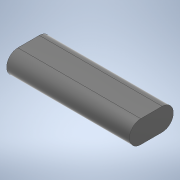
# Autodesk Inventor part: HX-2000MHT
Saved by Autodesk Inventor 2020 (Build 240168000, 168)
## iProperties
Created: 2019-11-07
Part Number: HX-2000MHT
Material: Generic
Document SubType Name: Modeling
Designer: maste
Density: 1 g/cm^3
Appearance: Smooth - Black
Author: maste
Autodesk Inventor part; units mm, degrees
ref_plane "YZ Plane" through (0, 0, 0) normal (1, 0, 0) x (0, 1, 0)
ref_plane "XZ Plane" through (0, 0, 0) normal (0, 1, 0) x (-1, 0, 0)
ref_plane "XY Plane" through (0, 0, 0) normal (0, 0, 1) x (1, 0, 0)
sketch "Sketch1" plane through (0, 0, 0) normal (1, 0, 0) x (0, 1, 0)
  line L0 (0, 0) -> (0, -46.5) construction
  line L1 (-11.9, -11.9) -> (-11.9, -34.6)
  line L2 (11.9, -34.6) -> (11.9, -11.9)
  arc A0 (11.9, -11.9) -> (-11.9, -11.9) centre (0, -11.9) ccw
  arc A1 (-11.9, -34.6) -> (11.9, -34.6) centre (0, -34.6) ccw
  point P0 (0, -23.25)
  dimension "d0" = 46.5
  dimension "d1" = 23.8
  constraints: 8 end point, 6 point on circle, 4 tangent, 2 centre point, 2 point on line, 1 midpoint, 1 parallel, 1 vertical
  measures "d0" distance of L0.start L0.end
  measures "d1" diameter of A1
extrude "Extrusion1" add sketch "Sketch1" along normal blind 130
body "Solid1"
